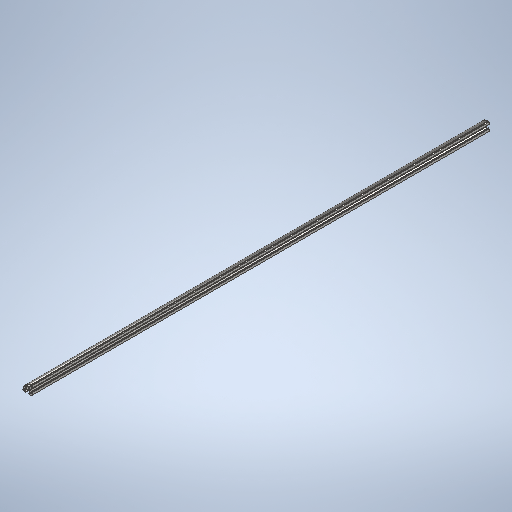
# Autodesk Inventor part: Ext_003
Saved by Autodesk Inventor 2025.2 (Build 292293000, 293)
## iProperties
Created: 2025-04-04
Part Number: Ext_003
Material: Aço galvanizado
Document SubType Name: Modeling
Designer: Formação
Density: 7.85 g/cm^3
Appearance: Galvanizado
Author: Formação
Autodesk Inventor part; units mm, degrees
ref_plane "YZ Plane" through (0, 0, 0) normal (1, 0, 0) x (0, 1, 0)
ref_plane "XZ Plane" through (0, 0, 0) normal (0, 1, 0) x (-1, 0, 0)
ref_plane "XY Plane" through (0, 0, 0) normal (0, 0, 1) x (1, 0, 0)
sketch "Esboço1" plane through (0, 0, 0) normal (0, 0, 1) x (1, 0, 0)
  line L0 (-10, 10) -> (10, 10) construction
  line L1 (10, 10) -> (10, -10) construction
  line L2 (10, -10) -> (-10, -10) construction
  line L3 (-10, -10) -> (-10, 10) construction
  line L4 (-10, 10) -> (10, -10) construction
  line L5 (10, 10) -> (-10, -10) construction
  circle A0 centre (0, 0) radius 2.5
  line L6 (10, 10) -> (1.7678, 1.7678) construction
  line L7 (1.7678, -1.7678) -> (10, -10) construction
  line L8 (-1.7678, -1.7678) -> (-10, -10) construction
  line L9 (-10, 10) -> (-1.7678, 1.7678) construction
  line L10 (4, 3.1) -> (4, -3.1) construction
  line L11 (-3.1, -5.0193) -> (3.1, -5.0193) construction
  line L12 (3.1, -5.0193) -> (10, -5.0193) construction
  line L13 (-3.1, -5.0193) -> (-10, -5.0193) construction
  line L14 (3.6312, 10) -> (10, 10) construction
  line L15 (3.6312, 10) -> (10, 10) construction
  line L16 (4, 3.1) -> (4, -3.1)
  line L17 (10, 9) -> (10, 4.1)
  line L18 (10, 4.1) -> (9, 4.1)
  line L19 (9, 4.1) -> (9, 3.1)
  line L20 (9, 3.1) -> (8, 3.1)
  line L21 (8, 3.1) -> (8, 6.1)
  arc A1 (8, 6.1) -> (7.275, 6.4381) centre (7.5586, 6.1) ccw
  line L22 (7.275, 6.4381) -> (4.0446, 3.2078)
  arc A2 (4.0446, 3.2078) -> (4, 3.1) centre (4.1524, 3.1) ccw
  line L23 (10, -9) -> (10, -4.1)
  line L24 (10, -4.1) -> (9, -4.1)
  line L25 (9, -4.1) -> (9, -3.1)
  line L26 (9, -3.1) -> (8, -3.1)
  line L27 (8, -3.1) -> (8, -6.1)
  arc A3 (7.275, -6.4381) -> (8, -6.1) centre (7.5586, -6.1) ccw
  arc A4 (4, -3.1) -> (4.0446, -3.2078) centre (4.1524, -3.1) ccw
  line L28 (7.275, -6.4381) -> (4.0446, -3.2078)
  arc A5 (9, -10) -> (10, -9) centre (9, -9) ccw
  arc A6 (10, 9) -> (9, 10) centre (9, 9) ccw
  line L29 (9, -10) -> (4.1, -10)
  line L30 (4.1, -10) -> (4.1, -9)
  line L31 (4.1, -9) -> (3.0767, -9)
  line L32 (3.0767, -9) -> (3.0767, -8)
  line L33 (3.0767, -8) -> (6.0767, -8)
  arc A7 (6.0767, -8) -> (6.4148, -7.275) centre (6.0767, -7.5586) ccw
  line L34 (-3.1233, -4) -> (3.0767, -4)
  arc A8 (3.1845, -4.0446) -> (3.0767, -4) centre (3.0767, -4.1524) ccw
  line L35 (3.1845, -4.0446) -> (6.4148, -7.275)
  arc A9 (-3.1233, -4) -> (-3.1913, -4.0281) centre (-3.1233, -4.0961) ccw
  line L36 (-9, -10) -> (-4.1, -10)
  line L37 (-4.1, -10) -> (-4.1, -9)
  line L38 (-4.1, -9) -> (-3.1, -9)
  line L39 (-3.1, -9) -> (-3.1, -8)
  line L40 (-3.1, -8) -> (-6.1, -8)
  arc A10 (-6.4381, -7.275) -> (-6.1, -8) centre (-6.1, -7.5586) ccw
  line L41 (-3.1913, -4.0281) -> (-6.4381, -7.275)
  arc A11 (-10, -9) -> (-9, -10) centre (-9, -9) ccw
  arc A12 (9, 10) -> (-10, -9) centre (9, -9) ccw
  line L42 (-3.7574, -3.2078) -> (-7.8245, -7.275)
  arc A13 (-3.7574, -3.2078) -> (-3.7127, -3.1) centre (-3.8651, -3.1) ccw
  line L43 (-3.7127, -3.1) -> (-3.7127, 3.1)
  line L44 (7.5486, 8.3855) -> (3.2062, 4.0431)
  arc A14 (-4.1418, 3.3001) -> (-8.8702, -6.8418) centre (9, -9) ccw
  arc A15 (-8.8702, -6.8418) -> (-7.8245, -7.275) centre (-8.2576, -6.8418) ccw
  arc A16 (-3.7127, 3.1) -> (-4.1418, 3.3001) centre (-3.9739, 3.1) ccw
  line L45 (3.0767, 4) -> (-3.1233, 4)
  arc A17 (3.0767, 4) -> (3.2062, 4.0431) centre (3.0984, 4.1509) ccw
  arc A18 (-3.3355, 4.5121) -> (-3.1233, 4) centre (-3.1233, 4.3) ccw
  arc A19 (7.1087, 9.1979) -> (-3.3355, 4.5121) centre (9, -9) ccw
  arc A20 (7.5486, 8.3855) -> (7.1087, 9.1979) centre (7.1604, 8.7006) ccw
  point P0 (4, 0)
  point P1 (4, 0)
  point P2 (8.5, 3.1)
  point P3 (7.7452, 6.5)
  point P4 (7.7452, -6.5)
  point P5 (9.7071, -9.7071)
  point P6 (9.7071, 9.7071)
  point P7 (-6.55, -10)
  point P8 (6.55, -10)
  point P9 (-4.435, 4.435)
  point P10 (-3.7127, 0)
  point P11 (-8.492, -7.4077)
  point P12 (-3.8635, 3.3367)
  point P13 (-0.0233, 4)
  point P14 (-0.0233, -4)
  point P15 (-3.4005, 4.1852)
  point P16 (7.6001, 8.9387)
  dimension "d0" = 20
  dimension "d1" = 20
  dimension "d3" = 5
  dimension "d34" = 1
  dimension "d35" = 1
  dimension "d36" = 2
  dimension "d37" = 130
  dimension "d38" = 6
  dimension "d39" = 6.9
  dimension "d41" = 4.9
  dimension "d42" = 4.9
  dimension "d47" = 45
  dimension "d49" = 3
  dimension "d51" = 13
  dimension "d52" = 4.9
  dimension "d56" = 90
  dimension "d57" = 1
  dimension "d58" = 3
  dimension "d59" = 130
  dimension "d62" = 45
  dimension "d63" = 1.2
  dimension "d64" = 45
  dimension "d65" = 4.9
  dimension "d66" = 1
  dimension "d67" = 1
  dimension "d68" = 1
  dimension "d70" = 3
  dimension "d71" = 130
  dimension "d73" = 90
  dimension "d74" = 19
  dimension "d75" = 6.2
  dimension "d80" = 45
  dimension "d94" = 18
  dimension "d96" = 135
  dimension "d98" = 130
  dimension "d99" = 10.7445
  dimension "d101" = 8
  dimension "d104" = 135
  dimension "d110" = 135
  dimension "d114" = 0.3
  constraints: 92 end point, 53 point on circle, 21 centre point, 18 tangent, 16 perpendicular, 14 point on line, 9 horizontal alignment, 9 midpoint, 8 horizontal, 7 equal length, 7 parallel, 7 vertical alignment, 5 equal radius, 4 vertical, 3 coincident, 2 collinear, 2 concentric, 1 other
  measures "d0" distance of L0.end L0.start
  measures "d1" distance of L1.end L0.end
  measures "d3" diameter of A0
  measures "d34" distance of L17.end L18.end
  measures "d35" distance of L18.end L19.end
  measures "d36" horizontal distance of L17.end L20.end
  measures "d38" horizontal distance of L17.end L10.end
  measures "d39" vertical distance of L0.end point (8.5, 3.1)
  measures "d41" distance of L17.end L17.start
  measures "d42" distance of L23.start L23.end
  measures "d49" distance of L21.end L20.end
  measures "d51" distance of point (7.745, -6.5) point (7.745, 6.5)
  measures "d52" distance of L29.start L29.end
  measures "d57" distance of L29.end L30.end
  measures "d58" distance of L32.end L33.end
  measures "d63" distance between parallel lines of L35 L28
  measures "d65" distance of L36.start L36.end
  measures "d66" distance of L2.end L36.start
  measures "d67" distance of L36.end L37.end
  measures "d68" distance of L37.end L38.end
  measures "d70" distance of L39.end L40.end
  measures "d74" radius of A12
  measures "d75" distance of L10.start L10.end
  measures "d94" radius of A14
  measures "d99" vertical distance of point (-8.492, -7.408) point (-3.864, 3.337)
  measures "d101" distance between parallel lines of L34 L45
  measures "d114" radius of A18
extrude "Extrusão1" add sketch "Esboço1" along normal mid plane 1000
